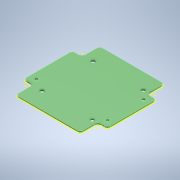
# Autodesk Inventor part: PCB
Saved by Autodesk Inventor 2021 (Build 250183000, 183)
## iProperties
Created: 2023-08-06
Part Number: PCB
Material: Generic
Document SubType Name: Modeling
Designer: michal
Density: 1 g/cm^3
Appearance: Smooth - Dark Forest Green
Author: michal
Autodesk Inventor part; units mm, degrees
ref_plane "YZ Plane" through (0, 0, 0) normal (1, 0, 0) x (0, 1, 0)
ref_plane "XZ Plane" through (0, 0, 0) normal (0, 1, 0) x (-1, 0, 0)
ref_plane "XY Plane" through (0, 0, 0) normal (0, 0, 1) x (1, 0, 0)
sketch "Sketch1" plane through (0, 0, 0) normal (0, 1, 0) x (-1, 0, 0)
  line L0 (-47.5, 47.5) -> (47.5, 47.5)
  line L1 (47.5, 47.5) -> (47.5, -47.5)
  line L2 (47.5, -47.5) -> (-47.5, -47.5)
  line L3 (-47.5, -47.5) -> (-47.5, 47.5)
  line L4 (-47.5, 47.5) -> (47.5, -47.5) construction
  line L5 (47.5, 47.5) -> (-47.5, -47.5) construction
  point P0 (0, 0)
  dimension "d0" = 95
  dimension "d1" = 95
  constraints: 12 end point, 2 midpoint, 2 parallel, 1 horizontal, 1 perpendicular
  measures "d0" distance of L1.end L2.end
  measures "d1" distance of L0.end L1.end
extrude "Extrusion1" add sketch "Sketch1" along normal blind 1.6
sketch "Sketch2" plane through (0, 1.6, 0) normal (0, 1, 0) x (1, 0, 0)
  line L0 (-47.5, -47.5) -> (47.5, -47.5) construction
  line L1 (-82.32, 0) -> (82.32, 0) construction
  line L2 (-47.5, 47.5) -> (-47.5, -47.5) projected
  line L3 (0, 73.5) -> (0, -73.5) construction
  point P0 (0, 0)
  point P1 (-40.395, -20.471)
  point P2 (40.395, -20.471)
  point P3 (-40.395, 20.471)
  point P4 (40.395, 20.471)
  dimension "d7" = 80.79
  dimension "d8" = 40.942
  constraints: 3 symmetric about line
  measures "d7" distance of point (40.395, -20.471) point (-40.395, -20.471)
  measures "d8" distance of point (-40.395, 20.471) point (-40.395, -20.471)
hole "Hole1" at (-40.395, 1.6, 20.471) at (40.395, 1.6, 20.471) at (40.395, 1.6, -20.471) direction (0, -1, 0) diameter 3 end through all counterbore diameter 6 counterbore depth 0.1
sketch "Sketch4" plane through (0, 1.6, 0) normal (0, 1, 0) x (1, 0, 0)
  line L0 (-47.5, 47.5) -> (-47.5, -47.5) projected
  line L1 (-47.5, -47.5) -> (-36.5, -47.5)
  line L2 (-36.5, -47.5) -> (-36.5, -27.5)
  line L3 (-36.5, -27.5) -> (-47.5, -27.5)
  line L4 (-47.5, -27.5) -> (-47.5, -47.5)
  line L5 (-47.5, -47.5) -> (47.5, -47.5) projected
  line L6 (47.5, -47.5) -> (36.5, -47.5)
  line L7 (36.5, -47.5) -> (36.5, -27.5)
  line L8 (36.5, -27.5) -> (47.5, -27.5)
  line L9 (47.5, -27.5) -> (47.5, -47.5)
  line L10 (-47.5, 47.5) -> (-36.5, 47.5)
  line L11 (-36.5, 47.5) -> (-36.5, 27.5)
  line L12 (-36.5, 27.5) -> (-47.5, 27.5)
  line L13 (-47.5, 27.5) -> (-47.5, 47.5)
  line L14 (47.5, 47.5) -> (-47.5, 47.5) projected
  line L15 (47.5, 47.5) -> (36.5, 47.5)
  line L16 (36.5, 47.5) -> (36.5, 27.5)
  line L17 (36.5, 27.5) -> (47.5, 27.5)
  line L18 (47.5, 27.5) -> (47.5, 47.5)
  point P0 (0, 0)
  point P1 (-47.5, -27.5)
  point P2 (-47.5, 27.5)
  dimension "d18" = 11
  dimension "d19" = 20
  dimension "d21" = 20
  dimension "d22" = 11
  dimension "d23" = 11
  dimension "d24" = 20
  dimension "d25" = 11
  dimension "d26" = 20
  constraints: 32 end point, 8 parallel, 4 horizontal, 4 perpendicular
  measures "d18" distance of L3.end L2.end
  measures "d19" distance of L2.end L1.end
  measures "d21" distance of L6.end L7.end
  measures "d22" distance of L16.end L17.end
  measures "d23" distance of L11.end L12.end
  measures "d24" distance of L15.end L16.end
  measures "d25" distance of L7.end L8.end
  measures "d26" distance of L10.end L11.end
extrude "Extrusion2" cut sketch "Sketch4" against normal blind 1.6
fillet "Fillet1" radius 4 4 edges at (36.5, 0.8, -27.5) (36.5, 0.8, 27.5) (-36.5, 0.8, 27.5) (-36.5, 0.8, -27.5)
fillet "Fillet2" radius 3 8 edges at (36.5, 0.8, 47.5) (-36.5, 0.8, 47.5) (-36.5, 0.8, -47.5) (36.5, 0.8, -47.5) (-47.5, 0.8, -27.5) (47.5, 0.8, -27.5) (47.5, 0.8, 27.5) (-47.5, 0.8, 27.5)
sketch "Sketch5" plane through (0, 0, 0) normal (0, -1, 0) x (1, 0, 0)
  ellipse E0 centre (-41.26, -32.3165) end of major axis (-44.0726, -35.129) minor radius 3.9748 (-37.2839, -32.3137) -> (-41.2573, -28.3403) ccw
  line L0 (-44.7377, -28.3403) -> (-41.2573, -28.3403)
  ellipse E1 centre (-44.7356, -25.3582) end of major axis (-46.845, -27.4676) minor radius 2.9811 (-47.1218, -27.1484) -> (-44.7377, -28.3403) ccw
  ellipse E2 centre (-44.7356, -25.3582) end of major axis (-46.845, -27.4676) minor radius 2.9811 (-47.7177, -25.3602) -> (-47.1218, -27.1484) ccw
  line L1 (-47.7177, -25.3602) -> (-47.7177, 25.3604)
  ellipse E3 centre (-44.7355, 25.3584) end of major axis (-42.6261, 23.249) minor radius 2.9811 (-46.5258, 27.7446) -> (-47.7177, 25.3604) ccw
  ellipse E4 centre (-44.7355, 25.3584) end of major axis (-42.6261, 23.249) minor radius 2.9811 (-44.7376, 28.3405) -> (-46.5258, 27.7446) ccw
  line L2 (-44.7376, 28.3405) -> (-41.2572, 28.3405)
  ellipse E5 centre (-41.26, 32.3167) end of major axis (-44.0725, 35.1292) minor radius 3.9748 (-41.2572, 28.3405) -> (-37.2838, 32.314) ccw
  line L3 (-37.2838, 44.7376) -> (-37.2838, 32.314)
  ellipse E6 centre (-34.3016, 44.7356) end of major axis (-36.411, 46.845) minor radius 2.9811 (-36.0919, 47.1218) -> (-37.2838, 44.7376) ccw
  ellipse E7 centre (-34.3016, 44.7356) end of major axis (-36.411, 46.845) minor radius 2.9811 (-34.3037, 47.7177) -> (-36.0919, 47.1218) ccw
  line L4 (-34.3037, 47.7177) -> (34.3036, 47.7176)
  ellipse E8 centre (34.3016, 44.7355) end of major axis (32.1921, 42.6261) minor radius 2.9811 (36.6877, 46.5257) -> (34.3036, 47.7176) ccw
  ellipse E9 centre (34.3016, 44.7355) end of major axis (32.1921, 42.6261) minor radius 2.9811 (37.2837, 44.7375) -> (36.6877, 46.5257) ccw
  line L5 (37.2837, 44.7375) -> (37.2837, 32.3139)
  ellipse E10 centre (41.2598, 32.3166) end of major axis (44.0724, 35.1291) minor radius 3.9748 (37.2837, 32.3139) -> (41.2571, 28.3404) ccw
  line L6 (44.7374, 28.3404) -> (41.2571, 28.3404)
  ellipse E11 centre (44.7354, 25.3583) end of major axis (42.626, 23.2489) minor radius 2.9811 (47.1216, 27.1485) -> (44.7374, 28.3404) ccw
  ellipse E12 centre (44.7354, 25.3583) end of major axis (42.626, 23.2489) minor radius 2.9811 (47.7175, 25.3603) -> (47.1216, 27.1485) ccw
  line L7 (47.7175, 25.3603) -> (47.7174, -25.3603)
  ellipse E13 centre (44.7353, -25.3583) end of major axis (46.8447, -27.4677) minor radius 2.9811 (46.5256, -27.7445) -> (47.7174, -25.3603) ccw
  ellipse E14 centre (44.7353, -25.3583) end of major axis (46.8447, -27.4677) minor radius 2.9811 (44.7374, -28.3404) -> (46.5256, -27.7445) ccw
  line L8 (44.7374, -28.3404) -> (41.257, -28.3404)
  ellipse E15 centre (41.2597, -32.3166) end of major axis (38.4472, -29.504) minor radius 3.9748 (41.257, -28.3404) -> (37.2836, -32.3139) ccw
  line L9 (37.2835, -44.7375) -> (37.2836, -32.3139)
  ellipse E16 centre (34.3014, -44.7355) end of major axis (32.192, -42.6261) minor radius 2.9811 (36.0917, -47.1217) -> (37.2835, -44.7375) ccw
  ellipse E17 centre (34.3014, -44.7355) end of major axis (32.192, -42.6261) minor radius 2.9811 (34.3035, -47.7176) -> (36.0917, -47.1217) ccw
  line L10 (34.3035, -47.7176) -> (-34.3038, -47.7175)
  ellipse E18 centre (-34.3018, -44.7354) end of major axis (-32.1924, -42.626) minor radius 2.9811 (-36.688, -46.5256) -> (-34.3038, -47.7175) ccw
  ellipse E19 centre (-34.3018, -44.7354) end of major axis (-32.1924, -42.626) minor radius 2.9811 (-37.2839, -44.7374) -> (-36.688, -46.5256) ccw
  line L11 (-37.2839, -44.7374) -> (-37.2839, -32.3137)
  arc A0 (29.8109, -43.3759) -> (29.8109, -37.4139) centre (29.8109, -40.3949) ccw
  arc A1 (29.8109, -37.4139) -> (29.8109, -43.3759) centre (29.8109, -40.3949) ccw
  arc A2 (-29.8112, -43.3759) -> (-29.8112, -37.4138) centre (-29.8112, -40.3948) ccw
  arc A3 (-29.8112, -37.4138) -> (-29.8112, -43.3759) centre (-29.8112, -40.3948) ccw
  arc A4 (-29.8111, 37.414) -> (-29.8111, 43.3761) centre (-29.8111, 40.395) ccw
  arc A5 (-29.8111, 43.3761) -> (-29.8111, 37.414) centre (-29.8111, 40.395) ccw
  arc A6 (29.811, 37.4139) -> (29.811, 43.376) centre (29.811, 40.3949) ccw
  arc A7 (29.811, 43.376) -> (29.811, 37.4139) centre (29.811, 40.3949) ccw
  arc A8 (40.3948, -23.4519) -> (40.3948, -17.4899) centre (40.3948, -20.4709) ccw
  arc A9 (40.3948, -17.4899) -> (40.3948, -23.4519) centre (40.3948, -20.4709) ccw
  arc A10 (40.3948, 17.4899) -> (40.3949, 23.4519) centre (40.3948, 20.4709) ccw
  arc A11 (40.3949, 23.4519) -> (40.3948, 17.4899) centre (40.3948, 20.4709) ccw
  arc A12 (-40.3951, -23.4518) -> (-40.3951, -17.4897) centre (-40.3951, -20.4708) ccw
  arc A13 (-40.3951, -17.4897) -> (-40.3951, -23.4518) centre (-40.3951, -20.4708) ccw
  arc A14 (-40.395, 17.49) -> (-40.395, 23.452) centre (-40.395, 20.471) ccw
  arc A15 (-40.395, 23.452) -> (-40.395, 17.49) centre (-40.395, 20.471) ccw
  line L12 (9.4429, -15.3772) -> (-9.4431, -15.3772) construction
  arc A16 (-9.4431, -15.3772) -> (-12.4251, -18.3592) centre (-9.4431, -18.3592) ccw construction
  line L13 (-12.4251, -18.3592) -> (-12.4251, -29.7902) construction
  arc A17 (-12.4251, -29.7902) -> (-9.4432, -32.7722) centre (-9.4431, -29.7902) ccw construction
  line L14 (-9.4432, -32.7722) -> (9.4428, -32.7722) construction
  arc A18 (9.4428, -32.7722) -> (12.4249, -29.7902) centre (9.4429, -29.7902) ccw construction
  line L15 (12.4249, -29.7902) -> (12.4249, -18.3592) construction
  arc A19 (12.4249, -18.3592) -> (9.4429, -15.3772) centre (9.4429, -18.3592) ccw construction
  arc A20 (11.9279, 31.7783) -> (11.9279, 21.8383) centre (11.9279, 26.8083) ccw construction
  arc A21 (11.9279, 21.8383) -> (11.9279, 31.7783) centre (11.9279, 26.8083) ccw construction
  arc A22 (-0.0001, 31.7783) -> (-0.0001, 21.8383) centre (-0.0001, 26.8083) ccw construction
  arc A23 (-0.0001, 21.8383) -> (-0.0001, 31.7783) centre (-0.0001, 26.8083) ccw construction
  arc A24 (-11.9281, 31.7783) -> (-11.9281, 21.8383) centre (-11.9281, 26.8083) ccw construction
  arc A25 (-11.9281, 21.8383) -> (-11.9281, 31.7783) centre (-11.9281, 26.8083) ccw construction
  arc A26 (14.9076, 45.7296) -> (14.9076, 39.7656) centre (14.9076, 42.7476) ccw construction
  arc A27 (14.9076, 39.7656) -> (14.9076, 45.7296) centre (14.9076, 42.7476) ccw construction
  arc A28 (31.7782, 16.3986) -> (31.7782, 10.4346) centre (31.7782, 13.4166) ccw construction
  arc A29 (31.7782, 10.4346) -> (31.7782, 16.3986) centre (31.7782, 13.4166) ccw construction
  arc A30 (31.7781, -10.4346) -> (31.7781, -16.3986) centre (31.7781, -13.4166) ccw construction
  arc A31 (31.7781, -16.3986) -> (31.7781, -10.4346) centre (31.7781, -13.4166) ccw construction
  arc A32 (14.9074, -39.7656) -> (14.9074, -45.7296) centre (14.9074, -42.7476) ccw construction
  arc A33 (14.9074, -45.7296) -> (14.9074, -39.7656) centre (14.9074, -42.7476) ccw construction
  arc A34 (-14.9077, 45.7297) -> (-14.9077, 39.7657) centre (-14.9077, 42.7477) ccw construction
  arc A35 (-14.9077, 39.7657) -> (-14.9077, 45.7297) centre (-14.9077, 42.7477) ccw construction
  arc A36 (-14.9078, -39.7655) -> (-14.9078, -45.7295) centre (-14.9078, -42.7475) ccw construction
  arc A37 (-14.9078, -45.7295) -> (-14.9078, -39.7655) centre (-14.9078, -42.7475) ccw construction
  arc A38 (-31.7784, -10.4345) -> (-31.7784, -16.3985) centre (-31.7784, -13.4165) ccw construction
  arc A39 (-31.7784, -16.3985) -> (-31.7784, -10.4345) centre (-31.7784, -13.4165) ccw construction
  arc A40 (-31.7783, 16.3987) -> (-31.7783, 10.4347) centre (-31.7783, 13.4167) ccw construction
  arc A41 (-31.7783, 10.4347) -> (-31.7783, 16.3987) centre (-31.7783, 13.4167) ccw construction
  arc A42 (41.3885, -3.5915) -> (41.3885, 3.5914) centre (40.3948, 0) ccw
  line L16 (41.3885, 3.5914) -> (41.3885, 7.9496)
  line L17 (41.3885, 7.9496) -> (39.4011, 7.9496)
  line L18 (39.4011, 7.9496) -> (39.4011, 3.5914)
  arc A43 (39.4011, 3.5914) -> (39.4011, -3.5914) centre (40.3948, 0) ccw
  line L19 (39.4011, -3.5914) -> (39.4011, -7.9496)
  line L20 (39.4011, -7.9496) -> (41.3885, -7.9496)
  line L21 (41.3885, -7.9496) -> (41.3885, -3.5915)
  arc A44 (-3.5916, -41.3886) -> (-0.0002, -44.1213) centre (-0.0002, -40.3949) ccw
  arc A45 (-0.0002, -44.1213) -> (3.5913, -41.3886) centre (-0.0002, -40.3949) ccw
  line L22 (3.5913, -41.3886) -> (7.9494, -41.3886)
  line L23 (7.9494, -41.3886) -> (7.9494, -39.4012)
  line L24 (7.9494, -39.4012) -> (3.5913, -39.4012)
  arc A46 (3.5913, -39.4012) -> (-0.0002, -36.6685) centre (-0.0002, -40.3949) ccw
  arc A47 (-0.0002, -36.6685) -> (-3.5916, -39.4012) centre (-0.0002, -40.3949) ccw
  line L25 (-3.5916, -39.4012) -> (-7.9498, -39.4012)
  line L26 (-7.9498, -39.4012) -> (-7.9498, -41.3886)
  line L27 (-7.9498, -41.3886) -> (-3.5916, -41.3886)
  arc A48 (-41.3887, 3.5916) -> (-41.3887, -3.5913) centre (-40.395, 0.0001) ccw
  line L28 (-41.3887, -3.5913) -> (-41.3887, -7.9495)
  line L29 (-41.3887, -7.9495) -> (-39.4013, -7.9495)
  line L30 (-39.4013, -7.9495) -> (-39.4013, -3.5913)
  arc A49 (-39.4013, -3.5913) -> (-39.4013, 3.5916) centre (-40.395, 0.0001) ccw
  line L31 (-39.4013, 3.5916) -> (-39.4013, 7.9497)
  line L32 (-39.4013, 7.9497) -> (-41.3887, 7.9497)
  line L33 (-41.3887, 7.9497) -> (-41.3887, 3.5916)
  arc A50 (3.5914, 41.3887) -> (0, 44.1214) centre (0, 40.395) ccw
  arc A51 (0, 44.1214) -> (-3.5915, 41.3887) centre (0, 40.395) ccw
  line L34 (-3.5915, 41.3887) -> (-7.9497, 41.3887)
  line L35 (-7.9497, 41.3887) -> (-7.9497, 39.4013)
  line L36 (-7.9497, 39.4013) -> (-3.5915, 39.4013)
  arc A52 (-3.5915, 39.4013) -> (-0.0001, 36.6686) centre (0, 40.395) ccw
  arc A53 (-0.0001, 36.6686) -> (3.5914, 39.4013) centre (0, 40.395) ccw
  line L37 (3.5914, 39.4013) -> (7.9496, 39.4013)
  line L38 (7.9496, 39.4013) -> (7.9496, 41.3887)
  line L39 (7.9496, 41.3887) -> (3.5914, 41.3887)
  spline S0 degree 3 poles (-0.0001, -3.4789) (0.3889, -3.4789) (0.7669, -3.4152) (1.1319, -3.2896) (1.1687, -3.277) (1.2053, -3.2637) (1.2418, -3.2497) (1.2547, -3.2448) (1.2666, -3.2402) (1.2805, -3.2347) (1.6979, -3.0694) (2.0707, -2.8307) (2.3946, -2.5235) (2.4165, -2.5026) (2.4383, -2.4814) (2.4598, -2.4599) (2.7882, -2.1317) (3.041, -1.7526) (3.2178, -1.3223) (3.2235, -1.3085) (3.2295, -1.2934) (3.2346, -1.2805) (3.3971, -0.8702) (3.4787, -0.4414) (3.4788, 0) (3.4789, 0.4277) (3.4027, 0.8417) (3.2497, 1.242) (3.2447, 1.2549) (3.2401, 1.2667) (3.2346, 1.2806) (3.0582, 1.7264) (2.7987, 2.121) (2.4598, 2.46) (2.1528, 2.7672) (1.8015, 3.0077) (1.4049, 3.1827) (1.3776, 3.1948) (1.35, 3.2065) (1.3223, 3.2179) (1.3084, 3.2236) (1.2933, 3.2297) (1.2805, 3.2348) (0.9196, 3.3776) (0.5476, 3.4574) (0.1611, 3.4753) (0.1075, 3.4778) (0.0538, 3.4791) (-0.0001, 3.4791) knots 0 0 0 0 0.110024 0.110024 0.110024 0.121094 0.121094 0.121094 0.125 0.125 0.125 0.242058 0.242058 0.242058 0.25 0.25 0.25 0.371094 0.371094 0.371094 0.375 0.375 0.375 0.5 0.5 0.5 0.621094 0.621094 0.621094 0.625 0.625 0.625 0.75 0.75 0.75 0.863286 0.863286 0.863286 0.871094 0.871094 0.871094 0.875 0.875 0.875 0.984792 0.984792 0.984792 1 1 1 1 construction
  spline S1 degree 3 poles (-0.0001, 3.4791) (-0.3891, 3.4791) (-0.7671, 3.4153) (-1.1321, 3.2897) (-1.1689, 3.2771) (-1.2055, 3.2638) (-1.2421, 3.2498) (-1.255, 3.2449) (-1.2668, 3.2403) (-1.2807, 3.2348) (-1.6981, 3.0695) (-2.0709, 2.8309) (-2.3948, 2.5236) (-2.4168, 2.5027) (-2.4385, 2.4815) (-2.4601, 2.46) (-2.7884, 2.1318) (-3.0412, 1.7527) (-3.218, 1.3225) (-3.2237, 1.3086) (-3.2298, 1.2935) (-3.2348, 1.2807) (-3.3973, 0.8703) (-3.4789, 0.4415) (-3.479, 0.0001) (-3.4791, -0.4276) (-3.4029, -0.8416) (-3.2499, -1.2418) (-3.245, -1.2548) (-3.2404, -1.2666) (-3.2348, -1.2805) (-3.0584, -1.7263) (-2.7989, -2.1209) (-2.4601, -2.4599) (-2.153, -2.7671) (-1.8017, -3.0075) (-1.4051, -3.1826) (-1.3778, -3.1947) (-1.3502, -3.2064) (-1.3225, -3.2178) (-1.3086, -3.2235) (-1.2935, -3.2296) (-1.2807, -3.2347) (-0.9199, -3.3775) (-0.5478, -3.4573) (-0.1613, -3.4752) (-0.1078, -3.4777) (-0.054, -3.4789) (-0.0001, -3.4789) knots 0 0 0 0 0.110024 0.110024 0.110024 0.121094 0.121094 0.121094 0.125 0.125 0.125 0.242058 0.242058 0.242058 0.25 0.25 0.25 0.371094 0.371094 0.371094 0.375 0.375 0.375 0.5 0.5 0.5 0.621094 0.621094 0.621094 0.625 0.625 0.625 0.75 0.75 0.75 0.863286 0.863286 0.863286 0.871094 0.871094 0.871094 0.875 0.875 0.875 0.984792 0.984792 0.984792 1 1 1 1 construction
  line L40 (-25.5065, -5.4684) -> (-28.5386, -5.4684) construction
  line L41 (-28.5386, -5.4684) -> (-26.2315, -10.4043) construction
  line L42 (-26.2315, -10.4043) -> (-28.327, -10.4043) construction
  line L43 (-28.327, -10.4043) -> (-28.327, -10.9684) construction
  line L44 (-28.327, -10.9684) -> (-25.436, -10.9684) construction
  line L45 (-25.436, -10.9684) -> (-27.7431, -6.0325) construction
  line L46 (-27.7431, -6.0325) -> (-25.5065, -6.0326) construction
  line L47 (-25.5065, -6.0326) -> (-25.5065, -5.4684) construction
  line L48 (-22.954, -8.0069) -> (-22.954, -5.4685) construction
  line L49 (-22.954, -5.4685) -> (-23.4476, -5.4685) construction
  line L50 (-23.4476, -5.4685) -> (-23.4476, -10.9685) construction
  line L51 (-23.4476, -10.9685) -> (-22.3689, -10.9685) construction
  spline S2 degree 3 poles (-22.3689, -10.9685) (-22.2947, -10.9684) (-22.1526, -10.9682) (-21.9488, -10.9635) (-21.7636, -10.9572) (-21.5976, -10.9484) (-21.4502, -10.938) (-21.322, -10.9235) (-21.2121, -10.9083) (-21.1463, -10.8929) (-21.1162, -10.8858) knots 0 0 0 0 0.176956 0.339055 0.486318 0.618781 0.735619 0.838742 0.926457 1 1 1 1 construction
  spline S3 degree 3 poles (-21.1162, -10.8858) (-21.0782, -10.8754) (-21.0031, -10.8549) (-20.8948, -10.8137) (-20.7918, -10.7648) (-20.6936, -10.7092) (-20.6021, -10.6442) (-20.5141, -10.574) (-20.4327, -10.4942) (-20.3569, -10.4072) (-20.2869, -10.3142) (-20.2281, -10.2134) (-20.1766, -10.1079) (-20.1345, -9.9963) (-20.1032, -9.8784) (-20.0799, -9.755) (-20.0651, -9.6261) (-20.0637, -9.538) (-20.0629, -9.4932) knots 0 0 0 0 0.062472 0.123472 0.183383 0.243116 0.302081 0.361286 0.42141 0.48249 0.544101 0.605721 0.667186 0.730025 0.794582 0.860367 0.928918 1 1 1 1 construction
  spline S4 degree 3 poles (-20.0629, -9.4932) (-20.0636, -9.448) (-20.0649, -9.3595) (-20.0804, -9.2301) (-20.1014, -9.1064) (-20.1336, -8.9887) (-20.1758, -8.8777) (-20.2253, -8.7718) (-20.285, -8.6726) (-20.3536, -8.58) (-20.4298, -8.4937) (-20.5135, -8.4144) (-20.6043, -8.3426) (-20.7018, -8.2781) (-20.807, -8.2223) (-20.9183, -8.1724) (-21.0367, -8.1305) (-21.1186, -8.1085) (-21.1603, -8.0973) knots 0 0 0 0 0.070119 0.137192 0.202016 0.264631 0.326117 0.38601 0.445812 0.505298 0.564633 0.624283 0.683902 0.743953 0.805388 0.868388 0.933084 1 1 1 1 construction
  spline S5 degree 3 poles (-21.1603, -8.0973) (-21.1948, -8.0899) (-21.2703, -8.0739) (-21.3946, -8.0559) (-21.5395, -8.0411) (-21.7044, -8.0273) (-21.8896, -8.0199) (-22.0949, -8.0114) (-22.3208, -8.0073) (-22.4784, -8.007) (-22.5606, -8.0069) knots 0 0 0 0 0.075172 0.164743 0.268011 0.385964 0.517799 0.663698 0.824417 1 1 1 1 construction
  line L52 (-22.5606, -8.0069) -> (-22.954, -8.0069) construction
  line L53 (-16.8052, -5.4685) -> (-16.8052, -10.4044) construction
  line L54 (-16.8052, -10.4044) -> (-17.6514, -10.4044) construction
  line L55 (-17.6514, -10.4044) -> (-17.3286, -10.9685) construction
  line L56 (-17.3286, -10.9685) -> (-16.3117, -10.9685) construction
  line L57 (-16.3117, -10.9685) -> (-16.3117, -5.4685) construction
  line L58 (-16.3117, -5.4685) -> (-16.8052, -5.4685) construction
  spline S6 degree 3 poles (-11.4972, -11.1095) (-11.4534, -11.1089) (-11.3663, -11.1077) (-11.2381, -11.0907) (-11.112, -11.0687) (-10.9902, -11.0336) (-10.8701, -10.9914) (-10.7549, -10.9359) (-10.6404, -10.8755) (-10.5319, -10.8017) (-10.4261, -10.7203) (-10.327, -10.6278) (-10.2319, -10.5268) (-10.1445, -10.4152) (-10.0611, -10.2945) (-9.9847, -10.1639) (-9.9138, -10.0235) (-9.8472, -9.874) (-9.7889, -9.7115) (-9.737, -9.537) (-9.6946, -9.3488) (-9.6594, -9.148) (-9.6322, -8.9336) (-9.6123, -8.7061) (-9.6018, -8.4654) (-9.5998, -8.3007) (-9.5988, -8.2163) knots 0 0 0 0 0.033788 0.067226 0.099841 0.132545 0.16513 0.198011 0.23128 0.265044 0.299216 0.334359 0.369695 0.406258 0.443804 0.482982 0.523085 0.565267 0.609343 0.656393 0.705887 0.758326 0.813833 0.872795 0.934723 1 1 1 1 construction
  spline S7 degree 3 poles (-9.5988, -8.2163) (-9.5999, -8.1322) (-9.6019, -7.9679) (-9.6121, -7.7282) (-9.6326, -7.5019) (-9.658, -7.2889) (-9.6935, -7.0889) (-9.7363, -6.9022) (-9.7851, -6.728) (-9.8443, -6.5676) (-9.9094, -6.4184) (-9.9802, -6.2791) (-10.0561, -6.1484) (-10.1383, -6.0275) (-10.2271, -5.9163) (-10.3221, -5.815) (-10.4222, -5.7219) (-10.5286, -5.6395) (-10.6381, -5.5653) (-10.7525, -5.5026) (-10.8691, -5.4484) (-10.9887, -5.404) (-11.1114, -5.3696) (-11.2376, -5.346) (-11.3664, -5.3293) (-11.4534, -5.3281) (-11.4972, -5.3274) knots 0 0 0 0 0.065069 0.127067 0.185532 0.240785 0.293004 0.342556 0.388955 0.432815 0.474671 0.514821 0.553655 0.591479 0.627861 0.663639 0.698823 0.733433 0.76763 0.801074 0.83425 0.86697 0.899712 0.932696 0.966173 1 1 1 1 construction
  spline S8 degree 3 poles (-11.4972, -5.3274) (-11.5405, -5.3282) (-11.6261, -5.3296) (-11.7528, -5.3446) (-11.8758, -5.3686) (-11.9957, -5.4023) (-12.1131, -5.4435) (-12.2264, -5.4971) (-12.3369, -5.5589) (-12.4442, -5.6293) (-12.5463, -5.71) (-12.6439, -5.7992) (-12.7344, -5.8992) (-12.8191, -6.0085) (-12.8985, -6.1267) (-12.9726, -6.2539) (-13.0407, -6.3905) (-13.103, -6.5371) (-13.1583, -6.6961) (-13.2069, -6.8688) (-13.2457, -7.0571) (-13.2786, -7.2601) (-13.305, -7.478) (-13.3234, -7.711) (-13.3345, -7.9587) (-13.3355, -8.1288) (-13.336, -8.2163) knots 0 0 0 0 0.033789 0.066625 0.099289 0.131367 0.163592 0.196113 0.228912 0.26217 0.296004 0.330232 0.365076 0.400968 0.437877 0.475966 0.51564 0.556675 0.600028 0.64669 0.696419 0.749772 0.80685 0.86743 0.931884 1 1 1 1 construction
  spline S9 degree 3 poles (-13.336, -8.2163) (-13.3355, -8.3044) (-13.3345, -8.4757) (-13.3234, -8.7252) (-13.3049, -8.9593) (-13.2795, -9.1779) (-13.2486, -9.3812) (-13.2074, -9.5686) (-13.1606, -9.7409) (-13.1063, -9.8987) (-13.045, -10.0442) (-12.9783, -10.18) (-12.9036, -10.306) (-12.8251, -10.424) (-12.7396, -10.5324) (-12.6491, -10.6323) (-12.5518, -10.7229) (-12.4486, -10.8043) (-12.3401, -10.8757) (-12.2295, -10.9389) (-12.1145, -10.991) (-11.9969, -11.0336) (-11.8763, -11.0684) (-11.7528, -11.0923) (-11.6261, -11.1073) (-11.5406, -11.1088) (-11.4972, -11.1095) knots 0 0 0 0 0.06859 0.133236 0.194298 0.251261 0.304491 0.354209 0.400451 0.443378 0.483979 0.523213 0.561001 0.597856 0.633471 0.668265 0.702638 0.736825 0.77043 0.803572 0.835925 0.86847 0.900854 0.933471 0.96626 1 1 1 1 construction
  spline S10 degree 3 poles (-6.3279, -8.5005) (-6.3706, -8.4996) (-6.4586, -8.4977) (-6.5936, -8.4839) (-6.7355, -8.4615) (-6.8837, -8.4307) (-7.0387, -8.3904) (-7.2001, -8.3422) (-7.3683, -8.2845) (-7.4816, -8.2409) (-7.5399, -8.2185) knots 0 0 0 0 0.102203 0.211023 0.3251 0.446502 0.573788 0.708901 0.850358 1 1 1 1 construction
  line L59 (-7.5399, -8.2185) -> (-6.9758, -10.9685) construction
  line L60 (-6.9758, -10.9685) -> (-4.7194, -10.9685) construction
  line L61 (-4.7194, -10.9685) -> (-4.7194, -10.4044) construction
  line L62 (-4.7194, -10.4044) -> (-6.5901, -10.4044) construction
  line L63 (-6.5901, -10.4044) -> (-6.8865, -8.9578) construction
  spline S11 degree 3 poles (-6.8865, -8.9578) (-6.8283, -8.9738) (-6.7155, -9.005) (-6.549, -9.0396) (-6.3909, -9.0604) (-6.2883, -9.0633) (-6.2387, -9.0646) knots 0 0 0 0 0.275068 0.532901 0.773973 1 1 1 1 construction
  spline S12 degree 3 poles (-6.2387, -9.0646) (-6.1773, -9.0633) (-6.0565, -9.0608) (-5.88, -9.0351) (-5.7107, -8.9979) (-5.5511, -8.9405) (-5.3986, -8.8704) (-5.2559, -8.7822) (-5.1209, -8.6792) (-4.9946, -8.5619) (-4.8806, -8.4315) (-4.7815, -8.2907) (-4.695, -8.1425) (-4.6275, -7.9836) (-4.5724, -7.817) (-4.5361, -7.6406) (-4.5119, -7.456) (-4.5092, -7.3298) (-4.5078, -7.2655) knots 0 0 0 0 0.0658 0.12938 0.190783 0.251293 0.31082 0.37037 0.43076 0.492598 0.554813 0.61609 0.676931 0.738289 0.800784 0.864793 0.931053 1 1 1 1 construction
  spline S13 degree 3 poles (-4.5078, -7.2655) (-4.5089, -7.2206) (-4.5109, -7.1316) (-4.5215, -6.9994) (-4.5419, -6.87) (-4.5689, -6.7436) (-4.605, -6.6202) (-4.6472, -6.499) (-4.6996, -6.3814) (-4.7578, -6.2669) (-4.8222, -6.1567) (-4.8946, -6.0535) (-4.9698, -5.955) (-5.052, -5.8641) (-5.1403, -5.7803) (-5.2341, -5.7034) (-5.3326, -5.632) (-5.4373, -5.5688) (-5.546, -5.5107) (-5.6601, -5.4631) (-5.7771, -5.4205) (-5.8987, -5.3865) (-6.0246, -5.3599) (-6.1549, -5.3419) (-6.2891, -5.3287) (-6.38, -5.3279) (-6.426, -5.3275) knots 0 0 0 0 0.044016 0.087438 0.130124 0.172561 0.214218 0.256302 0.298444 0.340536 0.382404 0.423614 0.464223 0.504052 0.543842 0.583548 0.623078 0.663214 0.703538 0.743927 0.784532 0.825742 0.867752 0.910741 0.954912 1 1 1 1 construction
  spline S14 degree 3 poles (-6.426, -5.3275) (-6.4808, -5.3285) (-6.5886, -5.3307) (-6.7466, -5.353) (-6.8985, -5.3851) (-7.0437, -5.4328) (-7.1815, -5.4951) (-7.314, -5.5693) (-7.4395, -5.6575) (-7.5572, -5.759) (-7.6653, -5.8706) (-7.7634, -5.9905) (-7.8496, -6.1189) (-7.9242, -6.2554) (-7.9879, -6.3998) (-8.0379, -6.5524) (-8.0782, -6.7125) (-8.0953, -6.8227) (-8.104, -6.8787) knots 0 0 0 0 0.06543 0.128725 0.190261 0.250757 0.310855 0.370776 0.431883 0.493799 0.556167 0.617293 0.678627 0.740678 0.80296 0.866786 0.932338 1 1 1 1 construction
  line L64 (-8.104, -6.8787) -> (-7.6104, -6.8787) construction
  spline S15 degree 3 poles (-7.6104, -6.8787) (-7.5982, -6.8263) (-7.5749, -6.7255) (-7.5236, -6.5839) (-7.4614, -6.4577) (-7.3858, -6.3461) (-7.2981, -6.2471) (-7.1962, -6.1597) (-7.0826, -6.0809) (-6.9562, -6.015) (-6.8227, -5.9595) (-6.6838, -5.9199) (-6.5414, -5.896) (-6.4455, -5.893) (-6.3973, -5.8916) knots 0 0 0 0 0.094686 0.181992 0.264373 0.341639 0.418558 0.496448 0.577307 0.661447 0.746668 0.831367 0.915207 1 1 1 1 construction
  spline S16 degree 3 poles (-6.3973, -5.8916) (-6.3503, -5.8929) (-6.2576, -5.8954) (-6.1211, -5.9148) (-5.9897, -5.9455) (-5.8632, -5.9884) (-5.7422, -6.0452) (-5.6268, -6.115) (-5.5155, -6.196) (-5.4111, -6.2886) (-5.3155, -6.3907) (-5.231, -6.4999) (-5.1606, -6.6164) (-5.1013, -6.7381) (-5.0563, -6.8665) (-5.0242, -7.0008) (-5.0053, -7.1415) (-5.0027, -7.2375) (-5.0014, -7.2864) knots 0 0 0 0 0.064204 0.126419 0.187672 0.248041 0.308337 0.36969 0.431725 0.49597 0.559779 0.622313 0.683925 0.745104 0.806749 0.869093 0.933293 1 1 1 1 construction
  spline S17 degree 3 poles (-5.0014, -7.2864) (-5.0024, -7.3305) (-5.0044, -7.4165) (-5.0213, -7.5428) (-5.0496, -7.6624) (-5.0898, -7.776) (-5.1401, -7.8832) (-5.2032, -7.9836) (-5.2764, -8.0783) (-5.3619, -8.1649) (-5.455, -8.2449) (-5.5579, -8.3128) (-5.6679, -8.3706) (-5.7854, -8.418) (-5.9103, -8.4557) (-6.0428, -8.4817) (-6.1829, -8.4973) (-6.2787, -8.4994) (-6.3279, -8.5005) knots 0 0 0 0 0.065358 0.127389 0.188368 0.24723 0.305649 0.363332 0.422657 0.482689 0.543308 0.604132 0.664984 0.727232 0.791447 0.858042 0.92703 1 1 1 1 construction
  spline S18 degree 3 poles (-1.6732, -5.8563) (-1.6751, -5.8261) (-1.6788, -5.7664) (-1.7028, -5.6796) (-1.7478, -5.6016) (-1.8059, -5.5315) (-1.8751, -5.4722) (-1.9543, -5.4293) (-2.0406, -5.403) (-2.1009, -5.3997) (-2.1315, -5.398) knots 0 0 0 0 0.126203 0.248871 0.371615 0.498901 0.627169 0.749175 0.872272 1 1 1 1 construction
  spline S19 degree 3 poles (-2.1315, -5.398) (-2.1622, -5.3996) (-2.2221, -5.4028) (-2.3081, -5.4298) (-2.3879, -5.4718) (-2.457, -5.5316) (-2.5156, -5.6012) (-2.5586, -5.6802) (-2.5847, -5.7662) (-2.5881, -5.826) (-2.5899, -5.8563) knots 0 0 0 0 0.127782 0.249465 0.372871 0.501195 0.628535 0.750593 0.873743 1 1 1 1 construction
  spline S20 degree 3 poles (-2.5899, -5.8563) (-2.5882, -5.8873) (-2.5849, -5.9479) (-2.5586, -6.0347) (-2.5155, -6.1135) (-2.4574, -6.1833) (-2.3874, -6.2417) (-2.3084, -6.2842) (-2.2219, -6.3094) (-2.1622, -6.3129) (-2.1315, -6.3146) knots 0 0 0 0 0.129097 0.252046 0.373905 0.501038 0.628171 0.751376 0.872426 1 1 1 1 construction
  spline S21 degree 3 poles (-2.1315, -6.3146) (-2.1009, -6.3128) (-2.0409, -6.3092) (-1.9541, -6.2848) (-1.8755, -6.2413) (-1.8055, -6.1834) (-1.7478, -6.1131) (-1.7028, -6.0352) (-1.6786, -5.9477) (-1.675, -5.8873) (-1.6732, -5.8563) knots 0 0 0 0 0.127519 0.249986 0.371792 0.49887 0.625948 0.748492 0.870959 1 1 1 1 construction
  line L65 (1.7255, -5.4685) -> (1.7255, -10.4044) construction
  line L66 (1.7255, -10.4044) -> (0.8794, -10.4044) construction
  line L67 (0.8794, -10.4044) -> (1.2022, -10.9685) construction
  line L68 (1.2022, -10.9685) -> (2.2191, -10.9685) construction
  line L69 (2.2191, -10.9685) -> (2.2191, -5.4685) construction
  line L70 (2.2191, -5.4685) -> (1.7255, -5.4685) construction
  spline S22 degree 3 poles (7.0336, -11.1095) (7.0774, -11.1089) (7.1644, -11.1077) (7.2927, -11.0907) (7.4187, -11.0688) (7.5406, -11.0336) (7.6607, -10.9915) (7.7759, -10.9359) (7.8903, -10.8755) (7.9988, -10.8018) (8.1046, -10.7203) (8.2038, -10.6278) (8.2989, -10.5269) (8.3863, -10.4152) (8.4697, -10.2946) (8.5461, -10.1639) (8.6169, -10.0235) (8.6836, -9.8741) (8.7419, -9.7115) (8.7937, -9.537) (8.8362, -9.3488) (8.8713, -9.148) (8.8986, -8.9337) (8.9185, -8.7062) (8.9289, -8.4654) (8.9309, -8.3008) (8.9319, -8.2163) knots 0 0 0 0 0.033788 0.067226 0.099841 0.132545 0.16513 0.198011 0.23128 0.265044 0.299216 0.334359 0.369695 0.406258 0.443804 0.482982 0.523085 0.565267 0.609343 0.656393 0.705887 0.758326 0.813833 0.872795 0.934723 1 1 1 1 construction
  spline S23 degree 3 poles (8.9319, -8.2163) (8.9309, -8.1322) (8.9289, -7.9679) (8.9187, -7.7282) (8.8981, -7.502) (8.8728, -7.2889) (8.8373, -7.0889) (8.7945, -6.9022) (8.7457, -6.728) (8.6865, -6.5676) (8.6214, -6.4185) (8.5506, -6.2791) (8.4747, -6.1485) (8.3925, -6.0275) (8.3036, -5.9163) (8.2086, -5.815) (8.1086, -5.7219) (8.0022, -5.6396) (7.8927, -5.5653) (7.7782, -5.5027) (7.6617, -5.4484) (7.542, -5.404) (7.4193, -5.3696) (7.2932, -5.346) (7.1644, -5.3294) (7.0774, -5.3281) (7.0336, -5.3275) knots 0 0 0 0 0.065069 0.127067 0.185532 0.240785 0.293004 0.342556 0.388955 0.432815 0.474671 0.514821 0.553655 0.591479 0.627861 0.663639 0.698823 0.733433 0.76763 0.801074 0.83425 0.86697 0.899712 0.932696 0.966173 1 1 1 1 construction
  spline S24 degree 3 poles (7.0336, -5.3275) (6.9902, -5.3282) (6.9047, -5.3296) (6.7779, -5.3446) (6.6549, -5.3686) (6.535, -5.4023) (6.4176, -5.4435) (6.3043, -5.4972) (6.1939, -5.559) (6.0866, -5.6294) (5.9844, -5.71) (5.8868, -5.7992) (5.7963, -5.8992) (5.7116, -6.0085) (5.6322, -6.1267) (5.5582, -6.254) (5.4901, -6.3905) (5.4278, -6.5371) (5.3725, -6.6961) (5.3239, -6.8688) (5.2851, -7.0572) (5.2522, -7.2601) (5.2258, -7.478) (5.2074, -7.7111) (5.1963, -7.9587) (5.1953, -8.1289) (5.1948, -8.2163) knots 0 0 0 0 0.033789 0.066625 0.099289 0.131367 0.163592 0.196113 0.228912 0.26217 0.296004 0.330232 0.365076 0.400968 0.437877 0.475966 0.51564 0.556675 0.600028 0.64669 0.696419 0.749772 0.80685 0.86743 0.931884 1 1 1 1 construction
  spline S25 degree 3 poles (5.1948, -8.2163) (5.1953, -8.3044) (5.1963, -8.4757) (5.2074, -8.7252) (5.2259, -8.9593) (5.2513, -9.1779) (5.2821, -9.3812) (5.3233, -9.5686) (5.3702, -9.7409) (5.4245, -9.8987) (5.4857, -10.0442) (5.5524, -10.18) (5.6272, -10.306) (5.7057, -10.424) (5.7911, -10.5324) (5.8816, -10.6323) (5.9789, -10.7229) (6.0822, -10.8043) (6.1906, -10.8757) (6.3013, -10.9389) (6.4162, -10.991) (6.5339, -11.0337) (6.6544, -11.0684) (6.778, -11.0923) (6.9047, -11.1074) (6.9902, -11.1088) (7.0336, -11.1095) knots 0 0 0 0 0.06859 0.133236 0.194298 0.251261 0.304491 0.354209 0.400451 0.443378 0.483979 0.523213 0.561001 0.597856 0.633471 0.668265 0.702638 0.736825 0.77043 0.803572 0.835925 0.86847 0.900854 0.933471 0.96626 1 1 1 1 construction
  spline S26 degree 3 poles (12.2028, -8.5006) (12.1602, -8.4996) (12.0722, -8.4978) (11.9372, -8.4839) (11.7953, -8.4615) (11.6471, -8.4307) (11.4921, -8.3905) (11.3307, -8.3422) (11.1625, -8.2845) (11.0492, -8.2409) (10.9909, -8.2185) knots 0 0 0 0 0.102203 0.211023 0.3251 0.446502 0.573788 0.708901 0.850358 1 1 1 1 construction
  line L71 (10.9909, -8.2185) -> (11.555, -10.9685) construction
  line L72 (11.555, -10.9685) -> (13.8114, -10.9685) construction
  line L73 (13.8114, -10.9685) -> (13.8114, -10.4044) construction
  line L74 (13.8114, -10.4044) -> (11.9406, -10.4044) construction
  line L75 (11.9406, -10.4044) -> (11.6443, -8.9578) construction
  spline S27 degree 3 poles (11.6443, -8.9578) (11.7025, -8.9739) (11.8153, -9.005) (11.9818, -9.0396) (12.1399, -9.0604) (12.2425, -9.0633) (12.2921, -9.0647) knots 0 0 0 0 0.275068 0.532901 0.773973 1 1 1 1 construction
  spline S28 degree 3 poles (12.2921, -9.0647) (12.3535, -9.0634) (12.4743, -9.0608) (12.6507, -9.0351) (12.82, -8.9979) (12.9797, -8.9405) (13.1321, -8.8705) (13.2749, -8.7822) (13.4099, -8.6792) (13.5362, -8.5619) (13.6502, -8.4315) (13.7493, -8.2907) (13.8358, -8.1426) (13.9033, -7.9837) (13.9583, -7.817) (13.9946, -7.6406) (14.0189, -7.456) (14.0216, -7.3298) (14.023, -7.2655) knots 0 0 0 0 0.0658 0.12938 0.190783 0.251293 0.31082 0.37037 0.43076 0.492598 0.554813 0.61609 0.676931 0.738289 0.800784 0.864793 0.931053 1 1 1 1 construction
  spline S29 degree 3 poles (14.023, -7.2655) (14.0219, -7.2207) (14.0198, -7.1316) (14.0093, -6.9994) (13.9889, -6.87) (13.9619, -6.7436) (13.9258, -6.6202) (13.8836, -6.499) (13.8311, -6.3814) (13.773, -6.2669) (13.7086, -6.1567) (13.6362, -6.0535) (13.5609, -5.955) (13.4787, -5.8641) (13.3905, -5.7804) (13.2967, -5.7035) (13.1982, -5.632) (13.0934, -5.5689) (12.9848, -5.5108) (12.8707, -5.4631) (12.7536, -5.4205) (12.6321, -5.3866) (12.5062, -5.36) (12.3758, -5.3419) (12.2417, -5.3287) (12.1507, -5.3279) (12.1048, -5.3275) knots 0 0 0 0 0.044016 0.087438 0.130124 0.172561 0.214218 0.256302 0.298444 0.340536 0.382404 0.423614 0.464223 0.504052 0.543842 0.583548 0.623078 0.663214 0.703538 0.743927 0.784532 0.825742 0.867752 0.910741 0.954912 1 1 1 1 construction
  spline S30 degree 3 poles (12.1048, -5.3275) (12.05, -5.3286) (11.9422, -5.3307) (11.7842, -5.353) (11.6323, -5.3852) (11.4871, -5.4328) (11.3493, -5.4952) (11.2168, -5.5693) (11.0913, -5.6575) (10.9736, -5.7591) (10.8655, -5.8706) (10.7674, -5.9905) (10.6812, -6.1189) (10.6065, -6.2554) (10.5429, -6.3998) (10.4929, -6.5524) (10.4525, -6.7125) (10.4355, -6.8228) (10.4268, -6.8788) knots 0 0 0 0 0.06543 0.128725 0.190261 0.250757 0.310855 0.370776 0.431883 0.493799 0.556167 0.617293 0.678627 0.740678 0.80296 0.866786 0.932338 1 1 1 1 construction
  line L76 (10.4268, -6.8788) -> (10.9204, -6.8788) construction
  spline S31 degree 3 poles (10.9204, -6.8788) (10.9325, -6.8263) (10.9559, -6.7255) (11.0072, -6.5839) (11.0694, -6.4577) (11.145, -6.3461) (11.2327, -6.2471) (11.3346, -6.1598) (11.4482, -6.0809) (11.5745, -6.015) (11.708, -5.9595) (11.847, -5.92) (11.9894, -5.896) (12.0852, -5.8931) (12.1334, -5.8916) knots 0 0 0 0 0.094686 0.181992 0.264373 0.341639 0.418558 0.496448 0.577307 0.661447 0.746668 0.831367 0.915207 1 1 1 1 construction
  spline S32 degree 3 poles (12.1334, -5.8916) (12.1805, -5.8929) (12.2732, -5.8954) (12.4097, -5.9148) (12.5411, -5.9455) (12.6676, -5.9884) (12.7886, -6.0452) (12.904, -6.115) (13.0153, -6.196) (13.1197, -6.2886) (13.2153, -6.3907) (13.2998, -6.4999) (13.3701, -6.6164) (13.4294, -6.7381) (13.4745, -6.8665) (13.5066, -7.0008) (13.5255, -7.1415) (13.528, -7.2375) (13.5294, -7.2864) knots 0 0 0 0 0.064204 0.126419 0.187672 0.248041 0.308337 0.36969 0.431725 0.49597 0.559779 0.622313 0.683925 0.745104 0.806749 0.869093 0.933293 1 1 1 1 construction
  spline S33 degree 3 poles (13.5294, -7.2864) (13.5284, -7.3305) (13.5264, -7.4165) (13.5095, -7.5428) (13.4812, -7.6625) (13.4409, -7.776) (13.3907, -7.8832) (13.3276, -7.9836) (13.2543, -8.0784) (13.1688, -8.1649) (13.0758, -8.2449) (12.9729, -8.3128) (12.8628, -8.3706) (12.7454, -8.418) (12.6205, -8.4557) (12.488, -8.4818) (12.3479, -8.4974) (12.2521, -8.4995) (12.2028, -8.5006) knots 0 0 0 0 0.065358 0.127389 0.188368 0.24723 0.305649 0.363332 0.422657 0.482689 0.543308 0.604132 0.664984 0.727232 0.791447 0.858042 0.92703 1 1 1 1 construction
  spline S34 degree 3 poles (16.8576, -5.8563) (16.8557, -5.8261) (16.852, -5.7664) (16.8279, -5.6796) (16.783, -5.6016) (16.7249, -5.5316) (16.6557, -5.4722) (16.5765, -5.4293) (16.4901, -5.403) (16.4299, -5.3997) (16.3992, -5.398) knots 0 0 0 0 0.126203 0.248871 0.371615 0.498901 0.627169 0.749175 0.872272 1 1 1 1 construction
  spline S35 degree 3 poles (16.3992, -5.398) (16.3686, -5.3996) (16.3086, -5.4028) (16.2226, -5.4299) (16.1429, -5.4718) (16.0737, -5.5317) (16.0152, -5.6013) (15.9722, -5.6802) (15.9461, -5.7662) (15.9426, -5.826) (15.9409, -5.8563) knots 0 0 0 0 0.127782 0.249465 0.372871 0.501195 0.628535 0.750593 0.873743 1 1 1 1 construction
  spline S36 degree 3 poles (15.9409, -5.8563) (15.9426, -5.8874) (15.9458, -5.948) (15.9722, -6.0347) (16.0152, -6.1135) (16.0734, -6.1833) (16.1433, -6.2417) (16.2224, -6.2843) (16.3089, -6.3095) (16.3686, -6.3129) (16.3992, -6.3147) knots 0 0 0 0 0.129097 0.252046 0.373905 0.501038 0.628171 0.751376 0.872426 1 1 1 1 construction
  spline S37 degree 3 poles (16.3992, -6.3147) (16.4299, -6.3128) (16.4899, -6.3093) (16.5767, -6.2848) (16.6553, -6.2413) (16.7253, -6.1834) (16.7829, -6.1132) (16.828, -6.0352) (16.8522, -5.9477) (16.8558, -5.8873) (16.8576, -5.8563) knots 0 0 0 0 0.127519 0.249986 0.371792 0.49887 0.625948 0.748492 0.870959 1 1 1 1 construction
  spline S38 degree 3 poles (20.5119, -5.3275) (20.4379, -5.3299) (20.2913, -5.3346) (20.0757, -5.3771) (19.8681, -5.4455) (19.6713, -5.5416) (19.4887, -5.661) (19.324, -5.8037) (19.1817, -5.97) (19.0622, -6.1562) (18.967, -6.3559) (18.8963, -6.5646) (18.8547, -6.7813) (18.849, -6.9282) (18.846, -7.0022) knots 0 0 0 0 0.084348 0.167078 0.249605 0.332974 0.416161 0.497811 0.580686 0.664926 0.749428 0.832484 0.915626 1 1 1 1 construction
  spline S39 degree 3 poles (18.846, -7.0022) (18.8479, -7.0588) (18.8517, -7.1745) (18.8782, -7.3496) (18.9207, -7.5288) (18.9683, -7.6809) (19.0186, -7.8054) (19.0605, -7.9059) (19.1127, -8.0092) (19.1682, -8.119) (19.2323, -8.2324) (19.3019, -8.3514) (19.3791, -8.474) (19.4332, -8.5572) (19.4608, -8.5997) knots 0 0 0 0 0.097818 0.199726 0.305276 0.415811 0.474472 0.537274 0.603657 0.674299 0.749834 0.828598 0.912378 1 1 1 1 construction
  line L77 (19.4608, -8.5997) -> (21.1024, -11.1095) construction
  line L78 (21.1024, -11.1095) -> (21.4826, -10.811) construction
  line L79 (21.4826, -10.811) -> (20.0293, -8.5887) construction
  spline S40 degree 3 poles (20.0293, -8.5887) (20.1261, -8.6041) (20.3148, -8.6342) (20.5058, -8.6392) (20.5989, -8.6416) knots 0 0 0 0 0.512659 1 1 1 1 construction
  spline S41 degree 3 poles (20.5989, -8.6416) (20.6548, -8.6401) (20.7649, -8.6371) (20.9264, -8.6144) (21.0817, -8.5785) (21.23, -8.5262) (21.3718, -8.4594) (21.5081, -8.3794) (21.6361, -8.2819) (21.7577, -8.1731) (21.8681, -8.0526) (21.9657, -7.9246) (22.0482, -7.7893) (22.1139, -7.6466) (22.1664, -7.4977) (22.2038, -7.3419) (22.2261, -7.1791) (22.2291, -7.0683) (22.2307, -7.0121) knots 0 0 0 0 0.065232 0.128407 0.19007 0.250947 0.311551 0.372869 0.435031 0.49908 0.5631 0.62552 0.686691 0.747683 0.80856 0.87074 0.93434 1 1 1 1 construction
  spline S42 degree 3 poles (22.2307, -7.0121) (22.2284, -6.9351) (22.224, -6.7837) (22.1801, -6.5631) (22.1124, -6.3531) (22.014, -6.1573) (21.8941, -5.9744) (21.7461, -5.8128) (21.5773, -5.6687) (21.3864, -5.5482) (21.1809, -5.4499) (20.9651, -5.3792) (20.741, -5.3357) (20.5889, -5.3303) (20.5119, -5.3275) knots 0 0 0 0 0.08595 0.16913 0.250406 0.33193 0.413348 0.494159 0.57601 0.660748 0.745776 0.830039 0.914025 1 1 1 1 construction
  spline S43 degree 3 poles (25.5644, -11.1095) (25.6081, -11.1089) (25.6952, -11.1077) (25.8235, -11.0907) (25.9495, -11.0688) (26.0714, -11.0336) (26.1914, -10.9915) (26.3066, -10.9359) (26.4211, -10.8755) (26.5296, -10.8018) (26.6354, -10.7203) (26.7346, -10.6278) (26.8296, -10.5269) (26.917, -10.4152) (27.0005, -10.2946) (27.0768, -10.1639) (27.1477, -10.0235) (27.2144, -9.8741) (27.2727, -9.7116) (27.3245, -9.537) (27.367, -9.3488) (27.4021, -9.148) (27.4294, -8.9337) (27.4492, -8.7062) (27.4597, -8.4654) (27.4617, -8.3008) (27.4627, -8.2163) knots 0 0 0 0 0.033788 0.067226 0.099841 0.132545 0.16513 0.198011 0.23128 0.265044 0.299216 0.334359 0.369695 0.406258 0.443804 0.482982 0.523085 0.565267 0.609343 0.656393 0.705887 0.758326 0.813833 0.872795 0.934723 1 1 1 1 construction
  spline S44 degree 3 poles (27.4627, -8.2163) (27.4617, -8.1322) (27.4596, -7.968) (27.4495, -7.7283) (27.4289, -7.502) (27.4036, -7.2889) (27.368, -7.089) (27.3252, -6.9022) (27.2765, -6.728) (27.2173, -6.5677) (27.1521, -6.4185) (27.0814, -6.2791) (27.0054, -6.1485) (26.9232, -6.0275) (26.8344, -5.9163) (26.7394, -5.815) (26.6394, -5.7219) (26.533, -5.6396) (26.4235, -5.5653) (26.309, -5.5027) (26.1925, -5.4484) (26.0728, -5.4041) (25.9501, -5.3697) (25.824, -5.346) (25.6952, -5.3294) (25.6081, -5.3281) (25.5644, -5.3275) knots 0 0 0 0 0.065069 0.127067 0.185532 0.240785 0.293004 0.342556 0.388955 0.432815 0.474671 0.514821 0.553655 0.591479 0.627861 0.663639 0.698823 0.733433 0.76763 0.801074 0.83425 0.86697 0.899712 0.932696 0.966173 1 1 1 1 construction
  spline S45 degree 3 poles (25.5644, -5.3275) (25.521, -5.3282) (25.4355, -5.3297) (25.3087, -5.3446) (25.1857, -5.3687) (25.0658, -5.4023) (24.9484, -5.4435) (24.8351, -5.4972) (24.7247, -5.559) (24.6173, -5.6294) (24.5152, -5.71) (24.4176, -5.7992) (24.3271, -5.8992) (24.2424, -6.0085) (24.163, -6.1267) (24.0889, -6.254) (24.0208, -6.3905) (23.9585, -6.5371) (23.9033, -6.6961) (23.8547, -6.8689) (23.8158, -7.0572) (23.7829, -7.2601) (23.7566, -7.478) (23.7382, -7.7111) (23.727, -7.9588) (23.726, -8.1289) (23.7255, -8.2163) knots 0 0 0 0 0.033789 0.066625 0.099289 0.131367 0.163592 0.196113 0.228912 0.26217 0.296004 0.330232 0.365076 0.400968 0.437877 0.475966 0.51564 0.556675 0.600028 0.64669 0.696419 0.749772 0.80685 0.86743 0.931884 1 1 1 1 construction
  spline S46 degree 3 poles (23.7255, -8.2163) (23.726, -8.3045) (23.727, -8.4757) (23.7382, -8.7252) (23.7567, -8.9593) (23.782, -9.178) (23.8129, -9.3812) (23.8541, -9.5686) (23.9009, -9.7409) (23.9552, -9.8988) (24.0165, -10.0443) (24.0832, -10.1801) (24.1579, -10.306) (24.2365, -10.4241) (24.3219, -10.5324) (24.4124, -10.6323) (24.5097, -10.7229) (24.613, -10.8043) (24.7214, -10.8757) (24.8321, -10.939) (24.947, -10.9911) (25.0646, -11.0337) (25.1852, -11.0685) (25.3087, -11.0924) (25.4354, -11.1074) (25.521, -11.1088) (25.5644, -11.1095) knots 0 0 0 0 0.06859 0.133236 0.194298 0.251261 0.304491 0.354209 0.400451 0.443378 0.483979 0.523213 0.561001 0.597856 0.633471 0.668265 0.702638 0.736825 0.77043 0.803572 0.835925 0.86847 0.900854 0.933471 0.96626 1 1 1 1 construction
  point P0 (0, 0)
  constraints: 20 other
sketch "Sketch6" plane through (0, 1.6, 0) normal (0, 1, 0) x (1, 0, 0)
  line L0 (31.5, 29) -> (-25.5, 29) construction
  line L1 (-25.5, 29) -> (-25.5, -29) construction
  line L2 (-25.5, -29) -> (31.5, -29) construction
  line L3 (31.5, -29) -> (31.5, 29) construction
  line L4 (31.5, 29) -> (-25.5, -29) construction
  line L5 (-25.5, 29) -> (31.5, -29) construction
  line L6 (-67.1987, 0) -> (67.1985, 0) construction
  line L7 (0, 67.1985) -> (0, -67.1986) construction
  point P0 (3, 0)
  dimension "d31" = 57
  dimension "d32" = 58
  dimension "d41" = 3
  constraints: 13 end point, 3 coincident, 2 parallel, 1 horizontal, 1 midpoint, 1 perpendicular, 1 point on line
  measures "d31" distance of L0.start L0.end
  measures "d32" distance of L0.end L1.end
  measures "d41" distance from line of point (3, 0) L7
hole "Hole2" at (-25.5, 1.6, 29) at (-25.5, 1.6, -29) at (31.5, 1.6, -29) at (31.5, 1.6, 29) direction (0, -1, 0) diameter 4.2 end through all
equation "\"d19\" = d21"
equation "\"d22\" = d18"
equation "\"d23\" = d18"
equation "\"d24\" = d19"
equation "\"d25\" = d18"
equation "\"d26\" = d21"
body "Solid1"
